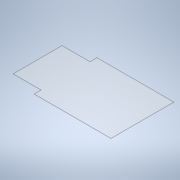
# Autodesk Inventor part: 2021 Underbelly
Saved by Autodesk Inventor 2021 (Build 250183000, 183)
## iProperties
Created: 2020-01-14
Part Number: 2021 Underbelly
Material: Polycarbonate, Clear
Document SubType Name: Modeling
Designer: aidan
Density: 1.2 g/cm^3
Appearance: Polycarbonate - Clear
Author: aidan
Autodesk Inventor part; units mm, degrees
ref_plane "YZ Plane" through (0, 0, 0) normal (1, 0, 0) x (0, 1, 0)
ref_plane "XZ Plane" through (0, 0, 0) normal (0, 1, 0) x (-1, 0, 0)
ref_plane "XY Plane" through (0, 0, 0) normal (0, 0, 1) x (1, 0, 0)
sketch "Sketch1" plane through (0, 0, 0) normal (0, 1, 0) x (-1, 0, 0)
  line L0 (374.9202, 193.7426) -> (-387.0798, 193.7426)
  line L1 (-387.0798, 193.7426) -> (-387.0798, -263.4574)
  line L2 (-387.0798, -263.4574) -> (374.9202, -263.4574)
  line L3 (374.9202, -263.4574) -> (374.9202, 193.7426)
  point P0 (0, 0)
  dimension "d0" = 457.2
  dimension "d1" = 762
  constraints: 8 end point, 2 parallel, 1 horizontal, 1 perpendicular
  measures "d0" distance of L2.end L0.start
  measures "d1" distance of L1.end L2.end
extrude "Extrusion1" add sketch "Sketch1" along normal blind 2.9972
sketch "Sketch3" plane through (0, 2.9972, 0) normal (0, 1, 0) x (1, 0, 0)
  line L0 (-374.9202, 212.6574) -> (-171.7202, 212.6574)
  line L1 (-171.7202, 212.6574) -> (-171.7202, 263.4574)
  line L2 (-171.7202, 263.4574) -> (-374.9202, 263.4574)
  line L3 (-374.9202, 263.4574) -> (-374.9202, 212.6574)
  line L4 (-374.9202, 263.4574) -> (-374.9202, -193.7426) projected
  line L5 (-374.9202, -193.7426) -> (-171.7202, -193.7426)
  line L6 (-171.7202, -193.7426) -> (-171.7202, -142.9426)
  line L7 (-171.7202, -142.9426) -> (-374.9202, -142.9426)
  line L8 (-374.9202, -142.9426) -> (-374.9202, -193.7426)
  line L9 (387.0798, 263.4574) -> (-374.9202, 263.4574) projected
  line L10 (387.0798, -193.7426) -> (387.0798, 263.4574) projected
  point P0 (0, 0)
  point P1 (-374.9202, -142.9426)
  dimension "d9" = 50.8
  dimension "d12" = 203.2
  constraints: 16 end point, 4 collinear, 4 parallel, 2 horizontal, 2 perpendicular, 1 point on line
  measures "d9" distance between parallel lines of L0 L2
  measures "d12" distance of L1.end L2.end
extrude "Extrusion3" cut sketch "Sketch3" against normal through all
body "Solid1"
